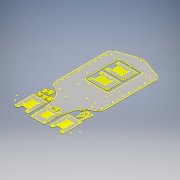
# Autodesk Inventor part: wjprep
Saved by Autodesk Inventor 2016 (Build 200138000, 138)
## iProperties
Created: 2015-08-04
Part Number: wjprep
Material: Generic
Document SubType Name: Modeling
Designer: brent
Density: 1 g/cm^3
Appearance: Default
Author: brent
Autodesk Inventor part; units mm, degrees
(part 1 of 6)
ref_plane "YZ Plane" through (0, 0, 0) normal (1, 0, 0) x (0, 1, 0)
ref_plane "XZ Plane" through (0, 0, 0) normal (0, 1, 0) x (-1, 0, 0)
ref_plane "XY Plane" through (0, 0, 0) normal (0, 0, 1) x (1, 0, 0)
sketch "Sketch1" plane through (0, 0, 0) normal (0, 1, 0) x (-1, 0, 0)
  line L0 (-14.0093, 246.3235) -> (-14.0093, 276.3235)
  arc A0 (-12.0093, 276.3235) -> (-14.0093, 276.3235) centre (-13.0093, 276.3235) ccw
  line L1 (-12.0093, 276.3235) -> (-12.0093, 246.3235)
  arc A1 (-14.0093, 246.3235) -> (-12.0093, 246.3235) centre (-13.0093, 246.3235) ccw
  line L2 (-14.9793, 220.366) -> (-14.9793, 228.674)
  arc A2 (-14.6363, 233.1974) -> (-14.9793, 228.674) centre (15.0207, 228.674) ccw
  arc A3 (-13.6478, 234.0466) -> (-14.6363, 233.1974) centre (-13.6478, 233.0466) ccw
  line L3 (-13.6478, 234.0466) -> (11.6292, 234.0466)
  arc A4 (12.6177, 233.1974) -> (11.6292, 234.0466) centre (11.6292, 233.0466) ccw
  arc A5 (12.9607, 228.674) -> (12.6177, 233.1974) centre (-17.0393, 228.674) ccw
  line L4 (12.9607, 228.674) -> (12.9607, 220.366)
  line L5 (9.9907, 246.3235) -> (9.9907, 276.3235)
  arc A6 (11.9907, 276.3235) -> (9.9907, 276.3235) centre (10.9907, 276.3235) ccw
  line L6 (11.9907, 276.3235) -> (11.9907, 246.3235)
  arc A7 (9.9907, 246.3235) -> (11.9907, 246.3235) centre (10.9907, 246.3235) ccw
  line L7 (5.9907, 246.3235) -> (5.9907, 276.3235)
  arc A8 (7.9907, 276.3235) -> (5.9907, 276.3235) centre (6.9907, 276.3235) ccw
  line L8 (7.9907, 276.3235) -> (7.9907, 246.3235)
  arc A9 (5.9907, 246.3235) -> (7.9907, 246.3235) centre (6.9907, 246.3235) ccw
  line L9 (1.9907, 246.3235) -> (1.9907, 276.3235)
  arc A10 (3.9907, 276.3235) -> (1.9907, 276.3235) centre (2.9907, 276.3235) ccw
  line L10 (3.9907, 276.3235) -> (3.9907, 246.3235)
  arc A11 (1.9907, 246.3235) -> (3.9907, 246.3235) centre (2.9907, 246.3235) ccw
  line L11 (-2.0093, 246.3235) -> (-2.0093, 276.3235)
  arc A12 (-0.0093, 276.3235) -> (-2.0093, 276.3235) centre (-1.0093, 276.3235) ccw
  line L12 (-0.0093, 276.3235) -> (-0.0093, 246.3235)
  arc A13 (-2.0093, 246.3235) -> (-0.0093, 246.3235) centre (-1.0093, 246.3235) ccw
  line L13 (-4.0093, 245.3235) -> (-5.0093, 245.3235)
  arc A14 (-6.0093, 246.3235) -> (-5.0093, 245.3235) centre (-5.0093, 246.3235) ccw
  line L14 (-6.0093, 246.3235) -> (-6.0093, 276.3235)
  arc A15 (-4.0093, 276.3235) -> (-6.0093, 276.3235) centre (-5.0093, 276.3235) ccw
  line L15 (-4.0093, 276.3235) -> (-4.0093, 245.3235)
  line L16 (-10.0093, 246.3235) -> (-10.0093, 276.3235)
  arc A16 (-8.0093, 276.3235) -> (-10.0093, 276.3235) centre (-9.0093, 276.3235) ccw
  line L17 (-8.0093, 276.3235) -> (-8.0093, 246.3235)
  arc A17 (-10.0093, 246.3235) -> (-8.0093, 246.3235) centre (-9.0093, 246.3235) ccw
  line L18 (-51.5093, -82.209) -> (-51.5093, 54.441)
  arc A18 (-48.3343, 57.616) -> (-51.5093, 54.441) centre (-48.3343, 54.441) ccw
  line L19 (-48.3343, 57.616) -> (46.3157, 57.616)
  arc A19 (49.4907, 54.441) -> (46.3157, 57.616) centre (46.3157, 54.441) ccw
  line L20 (49.4907, 54.441) -> (49.4907, -82.209)
  arc A20 (46.3157, -85.384) -> (49.4907, -82.209) centre (46.3157, -82.209) ccw
  line L21 (46.3157, -85.384) -> (-48.3343, -85.384)
  arc A21 (-51.5093, -82.209) -> (-48.3343, -85.384) centre (-48.3343, -82.209) ccw
  arc A22 (26.9307, 253.9347) -> (31.1366, 225.0046) centre (128.5307, 253.9347) ccw
  line L22 (26.9307, 253.9347) -> (26.9307, 296.8835)
  arc A23 (26.9307, 296.8835) -> (25.3432, 298.471) centre (25.3432, 296.8835) ccw
  line L23 (25.3432, 298.471) -> (-27.3618, 298.471)
  arc A24 (-27.3618, 298.471) -> (-28.9493, 296.8835) centre (-27.3618, 296.8835) ccw
  line L24 (-28.9493, 296.8835) -> (-28.9493, 253.9347)
  arc A25 (-33.1552, 225.0046) -> (-28.9493, 253.9347) centre (-130.5493, 253.9347) ccw
  line L25 (-101.6593, 123.6777) -> (-101.6593, -85.3463)
  arc A26 (-101.6593, -85.3463) -> (-88.4997, -104.1401) centre (-81.6593, -85.3463) ccw
  line L26 (-88.4997, -104.1401) -> (-18.1103, -129.7598)
  arc A27 (-18.1103, -129.7598) -> (16.0917, -129.7598) centre (-1.0093, -82.7751) ccw
  line L27 (16.0917, -129.7598) -> (86.4811, -104.1401)
  arc A28 (86.4811, -104.1401) -> (99.6407, -85.3463) centre (79.6407, -85.3463) ccw
  line L28 (99.6407, -85.3463) -> (99.6407, 123.6777)
  circle A29 centre (-17.0093, 277.3235) radius 1.25
  circle A30 centre (14.9907, 245.3235) radius 1.25
  circle A31 centre (-17.0093, 245.3235) radius 1.25
  circle A32 centre (14.9907, 277.3235) radius 1.25
  spline S0 degree 3 poles (31.1366, 225.0046) (32.3714, 220.8474) (33.4996, 216.6594) (35.5404, 208.2295) (36.4527, 203.9892) (37.256, 199.7275) knots 0 0 0 0 1.301003 1.301003 2.602005 2.602005 2.602005 2.602005
  line L29 (31.1366, 225.0046) -> (32.3714, 220.8474) construction
  line L30 (32.3714, 220.8474) -> (33.4996, 216.6594) construction
  line L31 (33.4996, 216.6594) -> (35.5404, 208.2295) construction
  line L32 (35.5404, 208.2295) -> (36.4527, 203.9892) construction
  line L33 (36.4527, 203.9892) -> (37.256, 199.7275) construction
  spline S1 degree 3 poles (68.3657, 155.8506) (67.5199, 156.3389) (66.0613, 157.226) (64.453, 158.2935) (63.2766, 159.1125) (62.5079, 159.667) (61.6622, 160.2983) (61.1095, 160.7227) (60.566, 161.1494) (60.2084, 161.4348) (59.6791, 161.8642) (59.161, 162.2937) (58.2156, 163.0982) (57.1975, 164.0023) (55.8635, 165.2517) (54.8824, 166.2209) (53.9184, 167.2151) (53.2845, 167.8903) (52.3477, 168.9211) (51.43, 169.9758) (50.092, 171.6007) (48.9455, 173.0897) (47.57, 175.003) (46.5174, 176.5739) (45.2648, 178.5838) (44.3148, 180.2271) (43.1951, 182.3209) (42.3549, 184.0258) (41.1802, 186.6232) (40.1209, 189.2718) (38.7567, 193.3177) (37.8697, 196.6666) (37.371, 199.1172) (37.256, 199.7275) knots 0.947472 0.947472 0.947472 0.947472 1.134532 1.274828 1.321593 1.415123 1.461888 1.532036 1.555419 1.602184 1.625566 1.695714 1.742479 1.882775 1.976305 2.1166 2.163365 2.256896 2.303661 2.443956 2.537487 2.724547 2.818077 3.005138 3.098668 3.285729 3.379259 3.56632 3.65985 3.940441 4.127501 4.501623 4.625555 4.625555 4.625555 4.625555
  line L34 (68.3657, 155.8506) -> (67.5199, 156.3389) construction
  line L35 (67.5199, 156.3389) -> (66.0613, 157.226) construction
  line L36 (66.0613, 157.226) -> (64.453, 158.2935) construction
  line L37 (64.453, 158.2935) -> (63.2766, 159.1125) construction
  line L38 (63.2766, 159.1125) -> (62.5079, 159.667) construction
  line L39 (62.5079, 159.667) -> (61.6622, 160.2983) construction
  line L40 (61.6622, 160.2983) -> (61.1095, 160.7227) construction
  line L41 (61.1095, 160.7227) -> (60.566, 161.1494) construction
  line L42 (60.566, 161.1494) -> (60.2084, 161.4348) construction
  line L43 (60.2084, 161.4348) -> (59.6791, 161.8642) construction
  line L44 (59.6791, 161.8642) -> (59.161, 162.2937) construction
  line L45 (59.161, 162.2937) -> (58.2156, 163.0982) construction
  line L46 (58.2156, 163.0982) -> (57.1975, 164.0023) construction
  line L47 (57.1975, 164.0023) -> (55.8635, 165.2517) construction
  line L48 (55.8635, 165.2517) -> (54.8824, 166.2209) construction
  line L49 (54.8824, 166.2209) -> (53.9184, 167.2151) construction
  line L50 (53.9184, 167.2151) -> (53.2845, 167.8903) construction
  line L51 (53.2845, 167.8903) -> (52.3477, 168.9211) construction
  line L52 (52.3477, 168.9211) -> (51.43, 169.9758) construction
  line L53 (51.43, 169.9758) -> (50.092, 171.6007) construction
  line L54 (50.092, 171.6007) -> (48.9455, 173.0897) construction
  line L55 (48.9455, 173.0897) -> (47.57, 175.003) construction
  line L56 (47.57, 175.003) -> (46.5174, 176.5739) construction
  line L57 (46.5174, 176.5739) -> (45.2648, 178.5838) construction
  line L58 (45.2648, 178.5838) -> (44.3148, 180.2271) construction
  line L59 (44.3148, 180.2271) -> (43.1951, 182.3209) construction
  line L60 (43.1951, 182.3209) -> (42.3549, 184.0258) construction
  line L61 (42.3549, 184.0258) -> (41.1802, 186.6232) construction
  line L62 (41.1802, 186.6232) -> (40.1209, 189.2718) construction
  line L63 (40.1209, 189.2718) -> (38.7567, 193.3177) construction
  line L64 (38.7567, 193.3177) -> (37.8697, 196.6666) construction
  line L65 (37.8697, 196.6666) -> (37.371, 199.1172) construction
  line L66 (37.371, 199.1172) -> (37.256, 199.7275) construction
  line L67 (87.4157, 144.852) -> (68.3657, 155.8506)
  spline S2 degree 3 poles (99.6407, 123.6777) (99.6407, 124.3721) (99.5814, 125.7789) (99.3501, 127.5553) (98.9988, 129.325) (98.6219, 130.7281) (98.0338, 132.4481) (97.4725, 133.7893) (96.6635, 135.4097) (95.9347, 136.6541) (95.034, 137.9833) (94.3922, 138.827) (93.7784, 139.5662) (93.4354, 139.9574) (93.1158, 140.3069) (92.9397, 140.4944) (92.7623, 140.6793) (92.6434, 140.8013) (92.4642, 140.9824) (92.2824, 141.1623) (92.005, 141.4297) (91.7534, 141.6647) (91.3686, 142.0128) (90.9741, 142.3548) (90.3647, 142.855) (89.8048, 143.2852) (89.0834, 143.8027) (88.3414, 144.2992) (87.7274, 144.6721) (87.4157, 144.852) knots 8.97392 8.97392 8.97392 8.97392 9.352631 9.731342 9.920698 10.29941 10.488765 10.867477 11.056832 11.435544 11.6249 11.908933 12.003611 12.145628 12.192967 12.263975 12.287645 12.334983 12.358653 12.429661 12.477 12.571678 12.619017 12.761034 12.855712 13.045067 13.139745 13.329101 13.518457 13.518457 13.518457 13.518457
  line L68 (99.6407, 123.6777) -> (99.6407, 124.3721) construction
  line L69 (99.6407, 124.3721) -> (99.5814, 125.7789) construction
  line L70 (99.5814, 125.7789) -> (99.3501, 127.5553) construction
  line L71 (99.3501, 127.5553) -> (98.9988, 129.325) construction
  line L72 (98.9988, 129.325) -> (98.6219, 130.7281) construction
  line L73 (98.6219, 130.7281) -> (98.0338, 132.4481) construction
  line L74 (98.0338, 132.4481) -> (97.4725, 133.7893) construction
  line L75 (97.4725, 133.7893) -> (96.6635, 135.4097) construction
  line L76 (96.6635, 135.4097) -> (95.9347, 136.6541) construction
  line L77 (95.9347, 136.6541) -> (95.034, 137.9833) construction
  line L78 (95.034, 137.9833) -> (94.3922, 138.827) construction
  line L79 (94.3922, 138.827) -> (93.7784, 139.5662) construction
  line L80 (93.7784, 139.5662) -> (93.4354, 139.9574) construction
  line L81 (93.4354, 139.9574) -> (93.1158, 140.3069) construction
  line L82 (93.1158, 140.3069) -> (92.9397, 140.4944) construction
  line L83 (92.9397, 140.4944) -> (92.7623, 140.6793) construction
  line L84 (92.7623, 140.6793) -> (92.6434, 140.8013) construction
  line L85 (92.6434, 140.8013) -> (92.4642, 140.9824) construction
  line L86 (92.4642, 140.9824) -> (92.2824, 141.1623) construction
  line L87 (92.2824, 141.1623) -> (92.005, 141.4297) construction
  line L88 (92.005, 141.4297) -> (91.7534, 141.6647) construction
  line L89 (91.7534, 141.6647) -> (91.3686, 142.0128) construction
  line L90 (91.3686, 142.0128) -> (90.9741, 142.3548) construction
  line L91 (90.9741, 142.3548) -> (90.3647, 142.855) construction
  line L92 (90.3647, 142.855) -> (89.8048, 143.2852) construction
  line L93 (89.8048, 143.2852) -> (89.0834, 143.8027) construction
  line L94 (89.0834, 143.8027) -> (88.3414, 144.2992) construction
  line L95 (88.3414, 144.2992) -> (87.7274, 144.6721) construction
  line L96 (87.7274, 144.6721) -> (87.4157, 144.852) construction
  spline S3 degree 3 poles (-89.4343, 144.852) (-89.746, 144.6721) (-90.36, 144.2992) (-91.102, 143.8027) (-91.8234, 143.2852) (-92.3833, 142.855) (-92.9927, 142.3548) (-93.3872, 142.0128) (-93.772, 141.6647) (-94.0236, 141.4297) (-94.301, 141.1623) (-94.4828, 140.9824) (-94.662, 140.8013) (-94.7809, 140.6793) (-94.9583, 140.4944) (-95.1344, 140.3069) (-95.454, 139.9574) (-95.797, 139.5662) (-96.4108, 138.827) (-97.0526, 137.9833) (-97.9533, 136.6541) (-98.6821, 135.4097) (-99.4911, 133.7893) (-100.0524, 132.4481) (-100.6405, 130.7281) (-101.0174, 129.325) (-101.3687, 127.5553) (-101.6, 125.7789) (-101.6593, 124.3721) (-101.6593, 123.6777) knots 0 0 0 0 0.189356 0.378711 0.473389 0.662745 0.757423 0.89944 0.946779 1.041456 1.088795 1.159804 1.183473 1.230812 1.254482 1.32549 1.372829 1.514846 1.609524 1.893557 2.082913 2.461624 2.65098 3.029691 3.219047 3.597759 3.787114 4.165826 4.544537 4.544537 4.544537 4.544537
  line L97 (-89.4343, 144.852) -> (-89.746, 144.6721) construction
  line L98 (-89.746, 144.6721) -> (-90.36, 144.2992) construction
  line L99 (-90.36, 144.2992) -> (-91.102, 143.8027) construction
  line L100 (-91.102, 143.8027) -> (-91.8234, 143.2852) construction
  line L101 (-91.8234, 143.2852) -> (-92.3833, 142.855) construction
  line L102 (-92.3833, 142.855) -> (-92.9927, 142.3548) construction
  line L103 (-92.9927, 142.3548) -> (-93.3872, 142.0128) construction
  line L104 (-93.3872, 142.0128) -> (-93.772, 141.6647) construction
  line L105 (-93.772, 141.6647) -> (-94.0236, 141.4297) construction
  line L106 (-94.0236, 141.4297) -> (-94.301, 141.1623) construction
  line L107 (-94.301, 141.1623) -> (-94.4828, 140.9824) construction
  line L108 (-94.4828, 140.9824) -> (-94.662, 140.8013) construction
  line L109 (-94.662, 140.8013) -> (-94.7809, 140.6793) construction
  line L110 (-94.7809, 140.6793) -> (-94.9583, 140.4944) construction
  line L111 (-94.9583, 140.4944) -> (-95.1344, 140.3069) construction
  line L112 (-95.1344, 140.3069) -> (-95.454, 139.9574) construction
  line L113 (-95.454, 139.9574) -> (-95.797, 139.5662) construction
  line L114 (-95.797, 139.5662) -> (-96.4108, 138.827) construction
  line L115 (-96.4108, 138.827) -> (-97.0526, 137.9833) construction
  line L116 (-97.0526, 137.9833) -> (-97.9533, 136.6541) construction
  line L117 (-97.9533, 136.6541) -> (-98.6821, 135.4097) construction
  line L118 (-98.6821, 135.4097) -> (-99.4911, 133.7893) construction
  line L119 (-99.4911, 133.7893) -> (-100.0524, 132.4481) construction
  line L120 (-100.0524, 132.4481) -> (-100.6405, 130.7281) construction
  line L121 (-100.6405, 130.7281) -> (-101.0174, 129.325) construction
  line L122 (-101.0174, 129.325) -> (-101.3687, 127.5553) construction
  line L123 (-101.3687, 127.5553) -> (-101.6, 125.7789) construction
  line L124 (-101.6, 125.7789) -> (-101.6593, 124.3721) construction
  line L125 (-101.6593, 124.3721) -> (-101.6593, 123.6777) construction
  line L126 (-70.3843, 155.8506) -> (-89.4343, 144.852)
  spline S4 degree 3 poles (-39.2746, 199.7275) (-39.3896, 199.1172) (-39.8883, 196.6666) (-40.7753, 193.3177) (-42.1395, 189.2718) (-43.1988, 186.6232) (-44.3735, 184.0258) (-45.2137, 182.3209) (-46.3334, 180.2271) (-47.2834, 178.5838) (-48.536, 176.5739) (-49.5886, 175.003) (-50.9641, 173.0897) (-52.1106, 171.6007) (-53.5973, 169.7952) (-54.8277, 168.3966) (-56.4124, 166.7087) (-57.7154, 165.4079) (-59.1326, 164.0805) (-59.9798, 163.3242) (-60.6639, 162.7326) (-61.0076, 162.44) (-61.3956, 162.115) (-61.6556, 161.9) (-61.9184, 161.6852) (-62.0947, 161.5421) (-62.3611, 161.3278) (-62.6299, 161.1138) (-63.1281, 160.7227) (-63.6808, 160.2982) (-64.5265, 159.667) (-65.2952, 159.1125) (-66.4717, 158.2935) (-68.0799, 157.226) (-69.5385, 156.3389) (-70.3843, 155.8506) knots 17.547092 17.547092 17.547092 17.547092 17.671024 18.045146 18.232206 18.512797 18.606327 18.793388 18.886918 19.073979 19.167509 19.35457 19.4481 19.63516 19.728691 19.915751 20.009282 20.196342 20.289872 20.406785 20.430168 20.476933 20.500316 20.535389 20.547081 20.570463 20.582155 20.617228 20.640611 20.710759 20.757524 20.851054 20.897819 21.038115 21.225175 21.225175 21.225175 21.225175
  line L127 (-39.2746, 199.7275) -> (-39.3896, 199.1172) construction
  line L128 (-39.3896, 199.1172) -> (-39.8883, 196.6666) construction
  line L129 (-39.8883, 196.6666) -> (-40.7753, 193.3177) construction
  line L130 (-40.7753, 193.3177) -> (-42.1395, 189.2718) construction
  line L131 (-42.1395, 189.2718) -> (-43.1988, 186.6232) construction
  line L132 (-43.1988, 186.6232) -> (-44.3735, 184.0258) construction
  line L133 (-44.3735, 184.0258) -> (-45.2137, 182.3209) construction
  line L134 (-45.2137, 182.3209) -> (-46.3334, 180.2271) construction
  line L135 (-46.3334, 180.2271) -> (-47.2834, 178.5838) construction
  line L136 (-47.2834, 178.5838) -> (-48.536, 176.5739) construction
  line L137 (-48.536, 176.5739) -> (-49.5886, 175.003) construction
  line L138 (-49.5886, 175.003) -> (-50.9641, 173.0897) construction
  line L139 (-50.9641, 173.0897) -> (-52.1106, 171.6007) construction
  line L140 (-52.1106, 171.6007) -> (-53.5973, 169.7952) construction
  line L141 (-53.5973, 169.7952) -> (-54.8277, 168.3966) construction
  line L142 (-54.8277, 168.3966) -> (-56.4124, 166.7087) construction
  line L143 (-56.4124, 166.7087) -> (-57.7154, 165.4079) construction
  line L144 (-57.7154, 165.4079) -> (-59.1326, 164.0805) construction
  line L145 (-59.1326, 164.0805) -> (-59.9798, 163.3242) construction
  line L146 (-59.9798, 163.3242) -> (-60.6639, 162.7326) construction
  line L147 (-60.6639, 162.7326) -> (-61.0076, 162.44) construction
  line L148 (-61.0076, 162.44) -> (-61.3956, 162.115) construction
  line L149 (-61.3956, 162.115) -> (-61.6556, 161.9) construction
  line L150 (-61.6556, 161.9) -> (-61.9184, 161.6852) construction
  line L151 (-61.9184, 161.6852) -> (-62.0947, 161.5421) construction
  line L152 (-62.0947, 161.5421) -> (-62.3611, 161.3278) construction
  line L153 (-62.3611, 161.3278) -> (-62.6299, 161.1138) construction
  line L154 (-62.6299, 161.1138) -> (-63.1281, 160.7227) construction
  line L155 (-63.1281, 160.7227) -> (-63.6808, 160.2982) construction
  line L156 (-63.6808, 160.2982) -> (-64.5265, 159.667) construction
  line L157 (-64.5265, 159.667) -> (-65.2952, 159.1125) construction
  line L158 (-65.2952, 159.1125) -> (-66.4717, 158.2935) construction
  line L159 (-66.4717, 158.2935) -> (-68.0799, 157.226) construction
  line L160 (-68.0799, 157.226) -> (-69.5385, 156.3389) construction
  line L161 (-69.5385, 156.3389) -> (-70.3843, 155.8506) construction
  spline S5 degree 3 poles (-39.2746, 199.7275) (-38.4713, 203.9892) (-37.559, 208.2295) (-35.5182, 216.6594) (-34.39, 220.8474) (-33.1552, 225.0046) knots 0 0 0 0 1.301003 1.301003 2.602005 2.602005 2.602005 2.602005
  line L162 (-39.2746, 199.7275) -> (-38.4713, 203.9892) construction
  line L163 (-38.4713, 203.9892) -> (-37.559, 208.2295) construction
  line L164 (-37.559, 208.2295) -> (-35.5182, 216.6594) construction
  line L165 (-35.5182, 216.6594) -> (-34.39, 220.8474) construction
  line L166 (-34.39, 220.8474) -> (-33.1552, 225.0046) construction
  spline S6 degree 3 poles (-24.3138, 291.486) (-24.3138, 291.8208) (-24.2469, 292.178) (-23.9748, 292.835) (-23.7696, 293.1349) (-23.296, 293.6085) (-22.9961, 293.8138) (-22.3389, 294.086) (-21.9817, 294.153) (-21.3119, 294.153) (-20.9547, 294.0861) (-20.2976, 293.8138) (-19.9976, 293.6085) (-19.5241, 293.1349) (-19.3189, 292.835) (-19.0467, 292.178) (-18.9798, 291.8208) (-18.9798, 291.1511) (-19.0467, 290.7939) (-19.3189, 290.1369) (-19.5241, 289.837) (-19.9976, 289.3634) (-20.2976, 289.1581) (-20.9547, 288.8859) (-21.3119, 288.819) (-21.9817, 288.819) (-22.3389, 288.8859) (-22.9961, 289.1581) (-23.296, 289.3635) (-23.7696, 289.8371) (-23.9748, 290.1369) (-24.2469, 290.7939) (-24.3138, 291.1511) (-24.3138, 291.486) knots -1.607821 -1.607821 -1.607821 -1.607821 -1.507361 -1.507361 -1.406901 -1.406901 -1.306377 -1.306377 -1.205854 -1.205854 -1.105342 -1.105342 -1.004829 -1.004829 -0.90437 -0.90437 -0.803911 -0.803911 -0.703451 -0.703451 -0.602992 -0.602992 -0.50248 -0.50248 -0.401967 -0.401967 -0.301444 -0.301444 -0.200921 -0.200921 -0.10046 -0.10046 0 0 0 0
  line L167 (-24.3138, 291.486) -> (-24.3138, 291.8208) construction
  line L168 (-24.3138, 291.8208) -> (-24.2469, 292.178) construction
  line L169 (-24.2469, 292.178) -> (-23.9748, 292.835) construction
  line L170 (-23.9748, 292.835) -> (-23.7696, 293.1349) construction
  line L171 (-23.7696, 293.1349) -> (-23.296, 293.6085) construction
  line L172 (-23.296, 293.6085) -> (-22.9961, 293.8138) construction
  line L173 (-22.9961, 293.8138) -> (-22.3389, 294.086) construction
  line L174 (-22.3389, 294.086) -> (-21.9817, 294.153) construction
  line L175 (-21.9817, 294.153) -> (-21.3119, 294.153) construction
  line L176 (-21.3119, 294.153) -> (-20.9547, 294.0861) construction
  line L177 (-20.9547, 294.0861) -> (-20.2976, 293.8138) construction
  line L178 (-20.2976, 293.8138) -> (-19.9976, 293.6085) construction
  line L179 (-19.9976, 293.6085) -> (-19.5241, 293.1349) construction
  line L180 (-19.5241, 293.1349) -> (-19.3189, 292.835) construction
  line L181 (-19.3189, 292.835) -> (-19.0467, 292.178) construction
  line L182 (-19.0467, 292.178) -> (-18.9798, 291.8208) construction
  line L183 (-18.9798, 291.8208) -> (-18.9798, 291.1511) construction
  line L184 (-18.9798, 291.1511) -> (-19.0467, 290.7939) construction
  line L185 (-19.0467, 290.7939) -> (-19.3189, 290.1369) construction
  line L186 (-19.3189, 290.1369) -> (-19.5241, 289.837) construction
  line L187 (-19.5241, 289.837) -> (-19.9976, 289.3634) construction
  line L188 (-19.9976, 289.3634) -> (-20.2976, 289.1581) construction
  line L189 (-20.2976, 289.1581) -> (-20.9547, 288.8859) construction
  line L190 (-20.9547, 288.8859) -> (-21.3119, 288.819) construction
  line L191 (-21.3119, 288.819) -> (-21.9817, 288.819) construction
  line L192 (-21.9817, 288.819) -> (-22.3389, 288.8859) construction
  line L193 (-22.3389, 288.8859) -> (-22.9961, 289.1581) construction
  line L194 (-22.9961, 289.1581) -> (-23.296, 289.3635) construction
  line L195 (-23.296, 289.3635) -> (-23.7696, 289.8371) construction
  line L196 (-23.7696, 289.8371) -> (-23.9748, 290.1369) construction
  line L197 (-23.9748, 290.1369) -> (-24.2469, 290.7939) construction
  line L198 (-24.2469, 290.7939) -> (-24.3138, 291.1511) construction
  line L199 (-24.3138, 291.1511) -> (-24.3138, 291.486) construction
  spline S7 degree 3 poles (16.9612, 291.486) (16.9612, 291.8208) (17.0281, 292.178) (17.3003, 292.835) (17.5055, 293.1349) (17.979, 293.6085) (18.279, 293.8138) (18.9361, 294.0861) (19.2933, 294.153) (19.9631, 294.153) (20.3203, 294.086) (20.9775, 293.8138) (21.2774, 293.6085) (21.751, 293.1349) (21.9562, 292.835) (22.2283, 292.178) (22.2952, 291.8208) (22.2952, 291.1511) (22.2283, 290.7939) (21.9562, 290.1369) (21.751, 289.8371) (21.2774, 289.3635) (20.9775, 289.1581) (20.3203, 288.8859) (19.9631, 288.819) (19.2933, 288.819) (18.9361, 288.8859) (18.279, 289.1581) (17.979, 289.3634) (17.5055, 289.837) (17.3003, 290.1369) (17.0281, 290.7939) (16.9612, 291.1511) (16.9612, 291.486) knots -1.607821 -1.607821 -1.607821 -1.607821 -1.507362 -1.507362 -1.406903 -1.406903 -1.30639 -1.30639 -1.205878 -1.205878 -1.105355 -1.105355 -1.004831 -1.004831 -0.904371 -0.904371 -0.803911 -0.803911 -0.70345 -0.70345 -0.60299 -0.60299 -0.502467 -0.502467 -0.401943 -0.401943 -0.301431 -0.301431 -0.200918 -0.200918 -0.100459 -0.100459 0 0 0 0
  line L200 (16.9612, 291.486) -> (16.9612, 291.8208) construction
  line L201 (16.9612, 291.8208) -> (17.0281, 292.178) construction
  line L202 (17.0281, 292.178) -> (17.3003, 292.835) construction
  line L203 (17.3003, 292.835) -> (17.5055, 293.1349) construction
  line L204 (17.5055, 293.1349) -> (17.979, 293.6085) construction
  line L205 (17.979, 293.6085) -> (18.279, 293.8138) construction
  line L206 (18.279, 293.8138) -> (18.9361, 294.0861) construction
  line L207 (18.9361, 294.0861) -> (19.2933, 294.153) construction
  line L208 (19.2933, 294.153) -> (19.9631, 294.153) construction
  line L209 (19.9631, 294.153) -> (20.3203, 294.086) construction
  line L210 (20.3203, 294.086) -> (20.9775, 293.8138) construction
  line L211 (20.9775, 293.8138) -> (21.2774, 293.6085) construction
  line L212 (21.2774, 293.6085) -> (21.751, 293.1349) construction
  line L213 (21.751, 293.1349) -> (21.9562, 292.835) construction
  line L214 (21.9562, 292.835) -> (22.2283, 292.178) construction
  line L215 (22.2283, 292.178) -> (22.2952, 291.8208) construction
  line L216 (22.2952, 291.8208) -> (22.2952, 291.1511) construction
  line L217 (22.2952, 291.1511) -> (22.2283, 290.7939) construction
  line L218 (22.2283, 290.7939) -> (21.9562, 290.1369) construction
  line L219 (21.9562, 290.1369) -> (21.751, 289.8371) construction
  line L220 (21.751, 289.8371) -> (21.2774, 289.3635) construction
  line L221 (21.2774, 289.3635) -> (20.9775, 289.1581) construction
  line L222 (20.9775, 289.1581) -> (20.3203, 288.8859) construction
  line L223 (20.3203, 288.8859) -> (19.9631, 288.819) construction
  line L224 (19.9631, 288.819) -> (19.2933, 288.819) construction
  line L225 (19.2933, 288.819) -> (18.9361, 288.8859) construction
  line L226 (18.9361, 288.8859) -> (18.279, 289.1581) construction
  line L227 (18.279, 289.1581) -> (17.979, 289.3634) construction
  line L228 (17.979, 289.3634) -> (17.5055, 289.837) construction
  line L229 (17.5055, 289.837) -> (17.3003, 290.1369) construction
  line L230 (17.3003, 290.1369) -> (17.0281, 290.7939) construction
  line L231 (17.0281, 290.7939) -> (16.9612, 291.1511) construction
  line L232 (16.9612, 291.1511) -> (16.9612, 291.486) construction
  circle A33 centre (-1.0093, -127.4103) radius 2.5527
  circle A34 centre (64.2282, 142.6982) radius 2.0193
  circle A35 centre (64.2282, -79.5518) radius 2.0193
  circle A36 centre (-66.2468, 31.5732) radius 2.0193
  circle A37 centre (-66.2468, -79.5518) radius 2.0193
  circle A38 centre (64.2282, 31.5732) radius 2.0193
  circle A39 centre (-66.2468, 142.6982) radius 2.0193
  circle A40 centre (45.4907, 86.566) radius 1.6
  circle A41 centre (-27.0093, 120.616) radius 1.6
  circle A42 centre (-59.0093, 73.616) radius 1.6
  circle A43 centre (-59.0093, 120.616) radius 1.6
  circle A44 centre (-27.0093, 73.616) radius 1.6
  circle A45 centre (24.9907, 156.566) radius 1.6
  circle A46 centre (4.4907, 86.566) radius 1.6
  spline S8 degree 3 poles (-24.3138, 227.986) (-24.3138, 228.3208) (-24.2469, 228.678) (-23.9748, 229.335) (-23.7696, 229.6349) (-23.296, 230.1085) (-22.9961, 230.3138) (-22.3389, 230.586) (-21.9817, 230.653) (-21.3119, 230.653) (-20.9547, 230.5861) (-20.2976, 230.3138) (-19.9976, 230.1085) (-19.5241, 229.6349) (-19.3189, 229.335) (-19.0467, 228.678) (-18.9798, 228.3208) (-18.9798, 227.6511) (-19.0467, 227.2939) (-19.3189, 226.6369) (-19.5241, 226.337) (-19.9976, 225.8634) (-20.2976, 225.6581) (-20.9547, 225.3859) (-21.3119, 225.319) (-21.9817, 225.319) (-22.3389, 225.3859) (-22.9961, 225.6581) (-23.296, 225.8635) (-23.7696, 226.3371) (-23.9748, 226.6369) (-24.2469, 227.2939) (-24.3138, 227.6511) (-24.3138, 227.986) knots -1.607821 -1.607821 -1.607821 -1.607821 -1.507361 -1.507361 -1.406901 -1.406901 -1.306377 -1.306377 -1.205854 -1.205854 -1.105342 -1.105342 -1.004829 -1.004829 -0.90437 -0.90437 -0.803911 -0.803911 -0.703451 -0.703451 -0.602992 -0.602992 -0.50248 -0.50248 -0.401967 -0.401967 -0.301444 -0.301444 -0.200921 -0.200921 -0.10046 -0.10046 0 0 0 0
  line L233 (-24.3138, 227.986) -> (-24.3138, 228.3208) construction
  line L234 (-24.3138, 228.3208) -> (-24.2469, 228.678) construction
  line L235 (-24.2469, 228.678) -> (-23.9748, 229.335) construction
  line L236 (-23.9748, 229.335) -> (-23.7696, 229.6349) construction
  line L237 (-23.7696, 229.6349) -> (-23.296, 230.1085) construction
  line L238 (-23.296, 230.1085) -> (-22.9961, 230.3138) construction
  line L239 (-22.9961, 230.3138) -> (-22.3389, 230.586) construction
  line L240 (-22.3389, 230.586) -> (-21.9817, 230.653) construction
  line L241 (-21.9817, 230.653) -> (-21.3119, 230.653) construction
  line L242 (-21.3119, 230.653) -> (-20.9547, 230.5861) construction
  line L243 (-20.9547, 230.5861) -> (-20.2976, 230.3138) construction
  line L244 (-20.2976, 230.3138) -> (-19.9976, 230.1085) construction
  line L245 (-19.9976, 230.1085) -> (-19.5241, 229.6349) construction
  line L246 (-19.5241, 229.6349) -> (-19.3189, 229.335) construction
  line L247 (-19.3189, 229.335) -> (-19.0467, 228.678) construction
  line L248 (-19.0467, 228.678) -> (-18.9798, 228.3208) construction
  line L249 (-18.9798, 228.3208) -> (-18.9798, 227.6511) construction
  line L250 (-18.9798, 227.6511) -> (-19.0467, 227.2939) construction
  line L251 (-19.0467, 227.2939) -> (-19.3189, 226.6369) construction
  line L252 (-19.3189, 226.6369) -> (-19.5241, 226.337) construction
  line L253 (-19.5241, 226.337) -> (-19.9976, 225.8634) construction
  line L254 (-19.9976, 225.8634) -> (-20.2976, 225.6581) construction
  line L255 (-20.2976, 225.6581) -> (-20.9547, 225.3859) construction
  line L256 (-20.9547, 225.3859) -> (-21.3119, 225.319) construction
  line L257 (-21.3119, 225.319) -> (-21.9817, 225.319) construction
  line L258 (-21.9817, 225.319) -> (-22.3389, 225.3859) construction
  line L259 (-22.3389, 225.3859) -> (-22.9961, 225.6581) construction
  line L260 (-22.9961, 225.6581) -> (-23.296, 225.8635) construction
  line L261 (-23.296, 225.8635) -> (-23.7696, 226.3371) construction
  line L262 (-23.7696, 226.3371) -> (-23.9748, 226.6369) construction
  line L263 (-23.9748, 226.6369) -> (-24.2469, 227.2939) construction
  line L264 (-24.2469, 227.2939) -> (-24.3138, 227.6511) construction
  line L265 (-24.3138, 227.6511) -> (-24.3138, 227.986) construction
  spline S9 degree 3 poles (16.9612, 227.986) (16.9612, 228.3208) (17.0281, 228.678) (17.3003, 229.335) (17.5055, 229.6349) (17.979, 230.1085) (18.279, 230.3138) (18.9361, 230.5861) (19.2933, 230.653) (19.9631, 230.653) (20.3203, 230.586) (20.9775, 230.3138) (21.2774, 230.1085) (21.751, 229.6349) (21.9562, 229.335) (22.2283, 228.678) (22.2952, 228.3208) (22.2952, 227.6511) (22.2283, 227.2939) (21.9562, 226.6369) (21.751, 226.3371) (21.2774, 225.8635) (20.9775, 225.6581) (20.3203, 225.3859) (19.9631, 225.319) (19.2933, 225.319) (18.9361, 225.3859) (18.279, 225.6581) (17.979, 225.8634) (17.5055, 226.337) (17.3003, 226.6369) (17.0281, 227.2939) (16.9612, 227.6511) (16.9612, 227.986) knots -1.607821 -1.607821 -1.607821 -1.607821 -1.507362 -1.507362 -1.406903 -1.406903 -1.30639 -1.30639 -1.205878 -1.205878 -1.105355 -1.105355 -1.004831 -1.004831 -0.904371 -0.904371 -0.803911 -0.803911 -0.70345 -0.70345 -0.60299 -0.60299 -0.502467 -0.502467 -0.401943 -0.401943 -0.301431 -0.301431 -0.200918 -0.200918 -0.100459 -0.100459 0 0 0 0
  line L266 (16.9612, 227.986) -> (16.9612, 228.3208) construction
  line L267 (16.9612, 228.3208) -> (17.0281, 228.678) construction
  line L268 (17.0281, 228.678) -> (17.3003, 229.335) construction
  line L269 (17.3003, 229.335) -> (17.5055, 229.6349) construction
  line L270 (17.5055, 229.6349) -> (17.979, 230.1085) construction
  line L271 (17.979, 230.1085) -> (18.279, 230.3138) construction
  line L272 (18.279, 230.3138) -> (18.9361, 230.5861) construction
  line L273 (18.9361, 230.5861) -> (19.2933, 230.653) construction
  line L274 (19.2933, 230.653) -> (19.9631, 230.653) construction
  line L275 (19.9631, 230.653) -> (20.3203, 230.586) construction
  line L276 (20.3203, 230.586) -> (20.9775, 230.3138) construction
  line L277 (20.9775, 230.3138) -> (21.2774, 230.1085) construction
  line L278 (21.2774, 230.1085) -> (21.751, 229.6349) construction
  line L279 (21.751, 229.6349) -> (21.9562, 229.335) construction
  line L280 (21.9562, 229.335) -> (22.2283, 228.678) construction
  line L281 (22.2283, 228.678) -> (22.2952, 228.3208) construction
  line L282 (22.2952, 228.3208) -> (22.2952, 227.6511) construction
  line L283 (22.2952, 227.6511) -> (22.2283, 227.2939) construction
  line L284 (22.2283, 227.2939) -> (21.9562, 226.6369) construction
  line L285 (21.9562, 226.6369) -> (21.751, 226.3371) construction
  line L286 (21.751, 226.3371) -> (21.2774, 225.8635) construction
  line L287 (21.2774, 225.8635) -> (20.9775, 225.6581) construction
  line L288 (20.9775, 225.6581) -> (20.3203, 225.3859) construction
  line L289 (20.3203, 225.3859) -> (19.9631, 225.319) construction
  line L290 (19.9631, 225.319) -> (19.2933, 225.319) construction
  line L291 (19.2933, 225.319) -> (18.9361, 225.3859) construction
  line L292 (18.9361, 225.3859) -> (18.279, 225.6581) construction
  line L293 (18.279, 225.6581) -> (17.979, 225.8634) construction
  line L294 (17.979, 225.8634) -> (17.5055, 226.337) construction
  line L295 (17.5055, 226.337) -> (17.3003, 226.6369) construction
  line L296 (17.3003, 226.6369) -> (17.0281, 227.2939) construction
  line L297 (17.0281, 227.2939) -> (16.9612, 227.6511) construction
  line L298 (16.9612, 227.6511) -> (16.9612, 227.986) construction
  spline S10 degree 3 poles (-8.6293, 214.016) (-9.4266, 214.016) (-10.2771, 214.1753) (-11.8416, 214.8234) (-12.5556, 215.3121) (-13.6832, 216.4396) (-14.1719, 217.1536) (-14.8199, 218.7181) (-14.9793, 219.5686) (-14.9793, 220.366) knots -0.956848 -0.956848 -0.956848 -0.956848 -0.71763 -0.71763 -0.478412 -0.478412 -0.239206 -0.239206 0 0 0 0
  line L299 (-8.6293, 214.016) -> (-9.4266, 214.016) construction
  line L300 (-9.4266, 214.016) -> (-10.2771, 214.1753) construction
  line L301 (-10.2771, 214.1753) -> (-11.8416, 214.8234) construction
  line L302 (-11.8416, 214.8234) -> (-12.5556, 215.3121) construction
  line L303 (-12.5556, 215.3121) -> (-13.6832, 216.4396) construction
  line L304 (-13.6832, 216.4396) -> (-14.1719, 217.1536) construction
  line L305 (-14.1719, 217.1536) -> (-14.8199, 218.7181) construction
  line L306 (-14.8199, 218.7181) -> (-14.9793, 219.5686) construction
  line L307 (-14.9793, 219.5686) -> (-14.9793, 220.366) construction
  line L308 (6.6107, 214.016) -> (-8.6293, 214.016)
  spline S11 degree 3 poles (12.9607, 220.366) (12.9607, 219.5686) (12.8014, 218.7182) (12.1533, 217.1537) (11.6647, 216.4397) (10.5371, 215.3121) (9.8231, 214.8234) (8.2586, 214.1753) (7.4081, 214.016) (6.6107, 214.016) knots -1.913649 -1.913649 -1.913649 -1.913649 -1.674451 -1.674451 -1.435253 -1.435253 -1.196027 -1.196027 -0.9568 -0.9568 -0.9568 -0.9568
  line L309 (12.9607, 220.366) -> (12.9607, 219.5686) construction
  line L310 (12.9607, 219.5686) -> (12.8014, 218.7182) construction
  line L311 (12.8014, 218.7182) -> (12.1533, 217.1537) construction
  line L312 (12.1533, 217.1537) -> (11.6647, 216.4397) construction
  line L313 (11.6647, 216.4397) -> (10.5371, 215.3121) construction
  line L314 (10.5371, 215.3121) -> (9.8231, 214.8234) construction
  line L315 (9.8231, 214.8234) -> (8.2586, 214.1753) construction
  line L316 (8.2586, 214.1753) -> (7.4081, 214.016) construction
  line L317 (7.4081, 214.016) -> (6.6107, 214.016) construction
  circle A47 centre (90.1157, -74.223) radius 2.5527
  circle A48 centre (90.1157, -29.773) radius 2.5527
  circle A49 centre (90.1157, 14.677) radius 2.5527
  circle A50 centre (90.1157, 59.127) radius 2.5527
  circle A51 centre (90.1157, 103.577) radius 2.5527
  circle A52 centre (90.1157, 125.802) radius 2.5527
  circle A53 centre (90.1157, 81.352) radius 2.5527
  circle A54 centre (90.1157, 36.902) radius 2.5527
  circle A55 centre (90.1157, -7.548) radius 2.5527
  circle A56 centre (90.1157, -51.998) radius 2.5527
  circle A57 centre (-92.1343, -7.548) radius 2.5527
  circle A58 centre (-92.1343, 36.902) radius 2.5527
  circle A59 centre (-92.1343, 81.352) radius 2.5527
  circle A60 centre (-92.1343, 125.802) radius 2.5527
  circle A61 centre (-92.1343, 103.577) radius 2.5527
  circle A62 centre (-92.1343, 59.127) radius 2.5527
  circle A63 centre (-92.1343, 14.677) radius 2.5527
  circle A64 centre (-92.1343, -29.773) radius 2.5527
  circle A65 centre (-92.1343, -74.223) radius 2.5527
  circle A66 centre (-92.1343, -51.998) radius 2.5527
  arc A67 (39.6262, 2.1558) -> (33.2762, 8.5058) centre (33.2762, 2.1558) ccw
  line L318 (33.2762, 8.5058) -> (31.9532, 8.5058)
  arc A68 (26.5806, 8.9908) -> (31.9532, 8.5058) centre (31.9532, 38.5058) ccw
  arc A69 (26.5806, 8.9908) -> (21.208, 9.4758) centre (21.208, -20.5242) ccw
  line L319 (21.208, 9.4758) -> (-15.6963, 9.4758)
  arc A70 (-15.6963, 11.4758) -> (-15.6963, 9.4758) centre (-15.6963, 10.4758) ccw
  line L320 (-15.6963, 11.4758) -> (23.3862, 11.4758)
  arc A71 (23.3862, 11.4758) -> (23.3862, 13.4758) centre (23.3862, 12.4758) ccw
  line L321 (23.3862, 13.4758) -> (-15.6963, 13.4758)
  arc A72 (-15.6963, 15.4758) -> (-15.6963, 13.4758) centre (-15.6963, 14.4758) ccw
  line L322 (-15.6963, 15.4758) -> (23.3862, 15.4758)
  arc A73 (23.3862, 15.4758) -> (23.3862, 17.4758) centre (23.3862, 16.4758) ccw
  line L323 (23.3862, 17.4758) -> (-15.6963, 17.4758)
  arc A74 (-15.6963, 19.4758) -> (-15.6963, 17.4758) centre (-15.6963, 18.4758) ccw
  line L324 (-15.6963, 19.4758) -> (23.3862, 19.4758)
  arc A75 (23.3862, 19.4758) -> (23.3862, 21.4758) centre (23.3862, 20.4758) ccw
  line L325 (23.3862, 21.4758) -> (-15.6963, 21.4758)
  arc A76 (-15.6963, 23.4758) -> (-15.6963, 21.4758) centre (-15.6963, 22.4758) ccw
  line L326 (-15.6963, 23.4758) -> (23.3862, 23.4758)
  arc A77 (23.3862, 23.4758) -> (23.3862, 25.4758) centre (23.3862, 24.4758) ccw
  line L327 (23.3862, 25.4758) -> (-15.6963, 25.4758)
  arc A78 (-15.6963, 27.4758) -> (-15.6963, 25.4758) centre (-15.6963, 26.4758) ccw
  line L328 (-15.6963, 27.4758) -> (23.3862, 27.4758)
  arc A79 (23.3862, 27.4758) -> (23.3862, 29.4758) centre (23.3862, 28.4758) ccw
  line L329 (23.3862, 29.4758) -> (-15.6963, 29.4758)
  arc A80 (-15.6963, 31.4758) -> (-15.6963, 29.4758) centre (-15.6963, 30.4758) ccw
  line L330 (-15.6963, 31.4758) -> (23.3862, 31.4758)
  arc A81 (23.3862, 31.4758) -> (23.3862, 33.4758) centre (23.3862, 32.4758) ccw
  line L331 (23.3862, 33.4758) -> (-15.6963, 33.4758)
  arc A82 (-15.6963, 35.4758) -> (-15.6963, 33.4758) centre (-15.6963, 34.4758) ccw
  line L332 (-15.6963, 35.4758) -> (21.208, 35.4758)
  arc A83 (21.208, 35.4758) -> (26.5806, 35.9608) centre (21.208, 65.4758) ccw
  arc A84 (31.9532, 36.4458) -> (26.5806, 35.9608) centre (31.9532, 6.4458) ccw
  line L333 (31.9532, 36.4458) -> (33.9112, 36.4458)
  arc A85 (33.9112, 36.4458) -> (40.2612, 42.7958) centre (33.9112, 42.7958) ccw
  line L334 (40.2612, 42.7958) -> (40.2612, 48.8283)
  arc A86 (40.2612, 48.8283) -> (38.6737, 50.4158) centre (38.6737, 48.8283) ccw
  line L335 (38.6737, 50.4158) -> (-36.2563, 50.4158)
  arc A87 (-36.2563, 50.4158) -> (-37.8438, 48.8283) centre (-36.2563, 48.8283) ccw
  line L336 (-37.8438, 48.8283) -> (-37.8438, -3.8731)
  arc A88 (-37.8438, -3.8731) -> (-36.2563, -5.4606) centre (-36.2563, -3.8731) ccw
  line L337 (-36.2563, -5.4606) -> (38.0387, -5.4606)
  arc A89 (38.0387, -5.4606) -> (39.6262, -3.8731) centre (38.0387, -3.8731) ccw
  line L338 (39.6262, -3.8731) -> (39.6262, 2.1558)
  spline S12 degree 3 poles (-30.8588, 40.4463) (-31.1937, 40.4463) (-31.5509, 40.5132) (-32.2079, 40.7853) (-32.5077, 40.9905) (-32.9814, 41.4641) (-33.1867, 41.764) (-33.4589, 42.4212) (-33.5258, 42.7784) (-33.5258, 43.4482) (-33.4589, 43.8054) (-33.1866, 44.4626) (-32.9813, 44.7625) (-32.5077, 45.236) (-32.2079, 45.4412) (-31.5509, 45.7133) (-31.1937, 45.7803) (-30.5239, 45.7803) (-30.1668, 45.7133) (-29.5098, 45.4412) (-29.2099, 45.236) (-28.7363, 44.7625) (-28.531, 44.4626) (-28.2587, 43.8054) (-28.1918, 43.4482) (-28.1918, 42.7784) (-28.2587, 42.4212) (-28.531, 41.764) (-28.7362, 41.4641) (-29.2099, 40.9905) (-29.5097, 40.7853) (-30.1668, 40.5132) (-30.524, 40.4463) (-30.8588, 40.4463) knots -1.607821 -1.607821 -1.607821 -1.607821 -1.507362 -1.507362 -1.406903 -1.406903 -1.30639 -1.30639 -1.205878 -1.205878 -1.105355 -1.105355 -1.004831 -1.004831 -0.904371 -0.904371 -0.803911 -0.803911 -0.70345 -0.70345 -0.60299 -0.60299 -0.502467 -0.502467 -0.401943 -0.401943 -0.301431 -0.301431 -0.200918 -0.200918 -0.100459 -0.100459 0 0 0 0
  line L339 (-30.8588, 40.4463) -> (-31.1937, 40.4463) construction
  line L340 (-31.1937, 40.4463) -> (-31.5509, 40.5132) construction
  line L341 (-31.5509, 40.5132) -> (-32.2079, 40.7853) construction
  line L342 (-32.2079, 40.7853) -> (-32.5077, 40.9905) construction
  line L343 (-32.5077, 40.9905) -> (-32.9814, 41.4641) construction
  line L344 (-32.9814, 41.4641) -> (-33.1867, 41.764) construction
  line L345 (-33.1867, 41.764) -> (-33.4589, 42.4212) construction
  line L346 (-33.4589, 42.4212) -> (-33.5258, 42.7784) construction
  line L347 (-33.5258, 42.7784) -> (-33.5258, 43.4482) construction
  line L348 (-33.5258, 43.4482) -> (-33.4589, 43.8054) construction
  line L349 (-33.4589, 43.8054) -> (-33.1866, 44.4626) construction
  line L350 (-33.1866, 44.4626) -> (-32.9813, 44.7625) construction
  line L351 (-32.9813, 44.7625) -> (-32.5077, 45.236) construction
  line L352 (-32.5077, 45.236) -> (-32.2079, 45.4412) construction
  line L353 (-32.2079, 45.4412) -> (-31.5509, 45.7133) construction
  line L354 (-31.5509, 45.7133) -> (-31.1937, 45.7803) construction
  line L355 (-31.1937, 45.7803) -> (-30.5239, 45.7803) construction
  line L356 (-30.5239, 45.7803) -> (-30.1668, 45.7133) construction
  line L357 (-30.1668, 45.7133) -> (-29.5098, 45.4412) construction
  line L358 (-29.5098, 45.4412) -> (-29.2099, 45.236) construction
  line L359 (-29.2099, 45.236) -> (-28.7363, 44.7625) construction
  line L360 (-28.7363, 44.7625) -> (-28.531, 44.4626) construction
  line L361 (-28.531, 44.4626) -> (-28.2587, 43.8054) construction
  line L362 (-28.2587, 43.8054) -> (-28.1918, 43.4482) construction
  line L363 (-28.1918, 43.4482) -> (-28.1918, 42.7784) construction
  line L364 (-28.1918, 42.7784) -> (-28.2587, 42.4212) construction
  line L365 (-28.2587, 42.4212) -> (-28.531, 41.764) construction
  line L366 (-28.531, 41.764) -> (-28.7362, 41.4641) construction
  line L367 (-28.7362, 41.4641) -> (-29.2099, 40.9905) construction
  line L368 (-29.2099, 40.9905) -> (-29.5097, 40.7853) construction
  line L369 (-29.5097, 40.7853) -> (-30.1668, 40.5132) construction
  line L370 (-30.1668, 40.5132) -> (-30.524, 40.4463) construction
  line L371 (-30.524, 40.4463) -> (-30.8588, 40.4463) construction
  spline S13 degree 3 poles (-30.8588, -0.8287) (-31.1937, -0.8287) (-31.5509, -0.7618) (-32.2079, -0.4897) (-32.5077, -0.2845) (-32.9813, 0.189) (-33.1866, 0.489) (-33.4589, 1.1461) (-33.5258, 1.5034) (-33.5258, 2.1731) (-33.4589, 2.5303) (-33.1867, 3.1875) (-32.9814, 3.4875) (-32.5077, 3.961) (-32.2079, 4.1662) (-31.5509, 4.4383) (-31.1937, 4.5053) (-30.524, 4.5053) (-30.1668, 4.4383) (-29.5097, 4.1662) (-29.2099, 3.961) (-28.7362, 3.4875) (-28.531, 3.1875) (-28.2587, 2.5303) (-28.1918, 2.1731) (-28.1918, 1.5034) (-28.2587, 1.1461) (-28.531, 0.489) (-28.7363, 0.189) (-29.2099, -0.2845) (-29.5098, -0.4897) (-30.1668, -0.7618) (-30.5239, -0.8287) (-30.8588, -0.8287) knots -1.607821 -1.607821 -1.607821 -1.607821 -1.507361 -1.507361 -1.406901 -1.406901 -1.306377 -1.306377 -1.205854 -1.205854 -1.105342 -1.105342 -1.004829 -1.004829 -0.90437 -0.90437 -0.803911 -0.803911 -0.703451 -0.703451 -0.602992 -0.602992 -0.50248 -0.50248 -0.401967 -0.401967 -0.301444 -0.301444 -0.200921 -0.200921 -0.10046 -0.10046 0 0 0 0
  line L372 (-30.8588, -0.8287) -> (-31.1937, -0.8287) construction
  line L373 (-31.1937, -0.8287) -> (-31.5509, -0.7618) construction
  line L374 (-31.5509, -0.7618) -> (-32.2079, -0.4897) construction
  line L375 (-32.2079, -0.4897) -> (-32.5077, -0.2845) construction
  line L376 (-32.5077, -0.2845) -> (-32.9813, 0.189) construction
  line L377 (-32.9813, 0.189) -> (-33.1866, 0.489) construction
  line L378 (-33.1866, 0.489) -> (-33.4589, 1.1461) construction
  line L379 (-33.4589, 1.1461) -> (-33.5258, 1.5034) construction
  line L380 (-33.5258, 1.5034) -> (-33.5258, 2.1731) construction
  line L381 (-33.5258, 2.1731) -> (-33.4589, 2.5303) construction
  line L382 (-33.4589, 2.5303) -> (-33.1867, 3.1875) construction
  line L383 (-33.1867, 3.1875) -> (-32.9814, 3.4875) construction
  line L384 (-32.9814, 3.4875) -> (-32.5077, 3.961) construction
  line L385 (-32.5077, 3.961) -> (-32.2079, 4.1662) construction
  line L386 (-32.2079, 4.1662) -> (-31.5509, 4.4383) construction
  line L387 (-31.5509, 4.4383) -> (-31.1937, 4.5053) construction
  line L388 (-31.1937, 4.5053) -> (-30.524, 4.5053) construction
  line L389 (-30.524, 4.5053) -> (-30.1668, 4.4383) construction
  line L390 (-30.1668, 4.4383) -> (-29.5097, 4.1662) construction
  line L391 (-29.5097, 4.1662) -> (-29.2099, 3.961) construction
  line L392 (-29.2099, 3.961) -> (-28.7362, 3.4875) construction
  line L393 (-28.7362, 3.4875) -> (-28.531, 3.1875) construction
  line L394 (-28.531, 3.1875) -> (-28.2587, 2.5303) construction
  line L395 (-28.2587, 2.5303) -> (-28.1918, 2.1731) construction
  line L396 (-28.1918, 2.1731) -> (-28.1918, 1.5034) construction
  line L397 (-28.1918, 1.5034) -> (-28.2587, 1.1461) construction
  line L398 (-28.2587, 1.1461) -> (-28.531, 0.489) construction
  line L399 (-28.531, 0.489) -> (-28.7363, 0.189) construction
  line L400 (-28.7363, 0.189) -> (-29.2099, -0.2845) construction
  line L401 (-29.2099, -0.2845) -> (-29.5098, -0.4897) construction
  line L402 (-29.5098, -0.4897) -> (-30.1668, -0.7618) construction
  line L403 (-30.1668, -0.7618) -> (-30.5239, -0.8287) construction
  line L404 (-30.5239, -0.8287) -> (-30.8588, -0.8287) construction
  spline S14 degree 3 poles (32.6412, -0.8287) (32.3063, -0.8287) (31.9491, -0.7618) (31.2921, -0.4897) (30.9923, -0.2845) (30.5187, 0.189) (30.3134, 0.489) (30.0411, 1.1461) (29.9742, 1.5034) (29.9742, 2.1731) (30.0411, 2.5303) (30.3133, 3.1875) (30.5186, 3.4875) (30.9923, 3.961) (31.2921, 4.1662) (31.9491, 4.4383) (32.3063, 4.5053) (32.976, 4.5053) (33.3332, 4.4383) (33.9903, 4.1662) (34.2901, 3.961) (34.7638, 3.4875) (34.969, 3.1875) (35.2413, 2.5303) (35.3082, 2.1731) (35.3082, 1.5034) (35.2413, 1.1461) (34.969, 0.489) (34.7637, 0.189) (34.2901, -0.2845) (33.9902, -0.4897) (33.3332, -0.7618) (32.9761, -0.8287) (32.6412, -0.8287) knots -1.607821 -1.607821 -1.607821 -1.607821 -1.507361 -1.507361 -1.406901 -1.406901 -1.306377 -1.306377 -1.205854 -1.205854 -1.105342 -1.105342 -1.004829 -1.004829 -0.90437 -0.90437 -0.803911 -0.803911 -0.703451 -0.703451 -0.602992 -0.602992 -0.50248 -0.50248 -0.401967 -0.401967 -0.301444 -0.301444 -0.200921 -0.200921 -0.10046 -0.10046 0 0 0 0
  line L405 (32.6412, -0.8287) -> (32.3063, -0.8287) construction
  line L406 (32.3063, -0.8287) -> (31.9491, -0.7618) construction
  line L407 (31.9491, -0.7618) -> (31.2921, -0.4897) construction
  line L408 (31.2921, -0.4897) -> (30.9923, -0.2845) construction
  line L409 (30.9923, -0.2845) -> (30.5187, 0.189) construction
  line L410 (30.5187, 0.189) -> (30.3134, 0.489) construction
  line L411 (30.3134, 0.489) -> (30.0411, 1.1461) construction
  line L412 (30.0411, 1.1461) -> (29.9742, 1.5034) construction
  line L413 (29.9742, 1.5034) -> (29.9742, 2.1731) construction
  line L414 (29.9742, 2.1731) -> (30.0411, 2.5303) construction
  line L415 (30.0411, 2.5303) -> (30.3133, 3.1875) construction
  line L416 (30.3133, 3.1875) -> (30.5186, 3.4875) construction
  line L417 (30.5186, 3.4875) -> (30.9923, 3.961) construction
  line L418 (30.9923, 3.961) -> (31.2921, 4.1662) construction
  line L419 (31.2921, 4.1662) -> (31.9491, 4.4383) construction
  line L420 (31.9491, 4.4383) -> (32.3063, 4.5053) construction
  line L421 (32.3063, 4.5053) -> (32.976, 4.5053) construction
  line L422 (32.976, 4.5053) -> (33.3332, 4.4383) construction
  line L423 (33.3332, 4.4383) -> (33.9903, 4.1662) construction
  line L424 (33.9903, 4.1662) -> (34.2901, 3.961) construction
  line L425 (34.2901, 3.961) -> (34.7638, 3.4875) construction
  line L426 (34.7638, 3.4875) -> (34.969, 3.1875) construction
  line L427 (34.969, 3.1875) -> (35.2413, 2.5303) construction
  line L428 (35.2413, 2.5303) -> (35.3082, 2.1731) construction
  line L429 (35.3082, 2.1731) -> (35.3082, 1.5034) construction
  line L430 (35.3082, 1.5034) -> (35.2413, 1.1461) construction
  line L431 (35.2413, 1.1461) -> (34.969, 0.489) construction
  line L432 (34.969, 0.489) -> (34.7637, 0.189) construction
  line L433 (34.7637, 0.189) -> (34.2901, -0.2845) construction
  line L434 (34.2901, -0.2845) -> (33.9902, -0.4897) construction
  line L435 (33.9902, -0.4897) -> (33.3332, -0.7618) construction
  line L436 (33.3332, -0.7618) -> (32.9761, -0.8287) construction
  line L437 (32.9761, -0.8287) -> (32.6412, -0.8287) construction
  spline S15 degree 3 poles (32.6412, 40.4463) (32.3063, 40.4463) (31.9491, 40.5132) (31.2921, 40.7853) (30.9923, 40.9905) (30.5186, 41.4641) (30.3133, 41.764) (30.0411, 42.4212) (29.9742, 42.7784) (29.9742, 43.4482) (30.0411, 43.8054) (30.3134, 44.4626) (30.5187, 44.7625) (30.9923, 45.236) (31.2921, 45.4412) (31.9491, 45.7133) (32.3063, 45.7803) (32.9761, 45.7803) (33.3332, 45.7133) (33.9902, 45.4412) (34.2901, 45.236) (34.7637, 44.7625) (34.969, 44.4626) (35.2413, 43.8054) (35.3082, 43.4482) (35.3082, 42.7784) (35.2413, 42.4212) (34.969, 41.764) (34.7638, 41.4641) (34.2901, 40.9905) (33.9903, 40.7853) (33.3332, 40.5132) (32.976, 40.4463) (32.6412, 40.4463) knots -1.607821 -1.607821 -1.607821 -1.607821 -1.507362 -1.507362 -1.406903 -1.406903 -1.30639 -1.30639 -1.205878 -1.205878 -1.105355 -1.105355 -1.004831 -1.004831 -0.904371 -0.904371 -0.803911 -0.803911 -0.70345 -0.70345 -0.60299 -0.60299 -0.502467 -0.502467 -0.401943 -0.401943 -0.301431 -0.301431 -0.200918 -0.200918 -0.100459 -0.100459 0 0 0 0
  line L438 (32.6412, 40.4463) -> (32.3063, 40.4463) construction
  line L439 (32.3063, 40.4463) -> (31.9491, 40.5132) construction
  line L440 (31.9491, 40.5132) -> (31.2921, 40.7853) construction
  line L441 (31.2921, 40.7853) -> (30.9923, 40.9905) construction
  line L442 (30.9923, 40.9905) -> (30.5186, 41.4641) construction
  line L443 (30.5186, 41.4641) -> (30.3133, 41.764) construction
  line L444 (30.3133, 41.764) -> (30.0411, 42.4212) construction
  line L445 (30.0411, 42.4212) -> (29.9742, 42.7784) construction
  line L446 (29.9742, 42.7784) -> (29.9742, 43.4482) construction
  line L447 (29.9742, 43.4482) -> (30.0411, 43.8054) construction
  line L448 (30.0411, 43.8054) -> (30.3134, 44.4626) construction